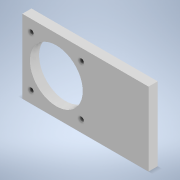
# Autodesk Inventor part: Stepper Plate
Saved by Autodesk Inventor 2020 (Build 240168000, 168)
## iProperties
Created: 2020-03-19
Part Number: Stepper Plate
Material: Generic
Document SubType Name: Modeling
Designer: DasNick
Density: 1 g/cm^3
Appearance: Default
Author: DasNick
Autodesk Inventor part; units mm, degrees
ref_plane "YZ Plane" through (0, 0, 0) normal (1, 0, 0) x (0, 1, 0)
ref_plane "XZ Plane" through (0, 0, 0) normal (0, 1, 0) x (-1, 0, 0)
ref_plane "XY Plane" through (0, 0, 0) normal (0, 0, 1) x (1, 0, 0)
sketch "Sketch1" plane through (0, 0, 0) normal (0, 0, 1) x (1, 0, 0)
  line L0 (-42.925, -19.7) -> (-38.525, -19.7) projected
  arc A0 (-38.525, -28.9) -> (-38.525, -19.7) centre (-38.525, -24.3) ccw projected
  line L1 (-38.525, -28.9) -> (-42.925, -28.9) projected
  line L2 (-42.925, -37.425) -> (-42.925, -28.9) projected
  arc A1 (-42.925, -37.425) -> (-37.425, -42.925) centre (-37.425, -37.425) ccw projected
  line L3 (19.7, -42.925) -> (-37.425, -42.925) projected
  line L4 (19.7, -42.925) -> (19.7, -38.525) projected
  arc A2 (28.9, -38.525) -> (19.7, -38.525) centre (24.3, -38.525) ccw projected
  line L5 (28.9, -38.525) -> (28.9, -42.925) projected
  line L6 (37.425, -42.925) -> (28.9, -42.925) projected
  arc A3 (37.425, -42.925) -> (42.925, -37.425) centre (37.425, -37.425) ccw projected
  line L7 (42.925, 19.7) -> (42.925, -37.425) projected
  line L8 (42.925, 19.7) -> (38.525, 19.7) projected
  arc A4 (38.525, 28.9) -> (38.525, 19.7) centre (38.525, 24.3) ccw projected
  line L9 (38.525, 28.9) -> (42.925, 28.9) projected
  line L10 (42.925, 37.425) -> (42.925, 28.9) projected
  arc A5 (42.925, 37.425) -> (37.425, 42.925) centre (37.425, 37.425) ccw projected
  line L11 (-19.7, 42.925) -> (37.425, 42.925) projected
  line L12 (-19.7, 42.925) -> (-19.7, 38.525) projected
  arc A6 (-28.9, 38.525) -> (-19.7, 38.525) centre (-24.3, 38.525) ccw projected
  line L13 (-28.9, 38.525) -> (-28.9, 42.925) projected
  line L14 (-37.425, 42.925) -> (-28.9, 42.925) projected
  arc A7 (-37.425, 42.925) -> (-42.925, 37.425) centre (-37.425, 37.425) ccw projected
  line L15 (-42.925, -19.7) -> (-42.925, 37.425) projected
  circle A8 centre (34.75, -34.75) radius 3.3 projected
  circle A9 centre (-34.75, -34.75) radius 3.3 projected
  circle A10 centre (34.75, 34.75) radius 3.3 projected
  circle A11 centre (-34.75, 34.75) radius 3.3 projected
  circle A12 centre (0, 0) radius 36.5125 projected
  line L16 (127.3875, 50.7471) -> (127.3875, -50.8529) projected
  line L17 (127.3875, 50.7471) -> (-47.0237, 50.7471)
  line L18 (-47.0237, 50.7471) -> (-47.0237, -50.8529)
  line L19 (-47.0237, -50.8529) -> (127.3875, -50.8529)
  point P0 (0, 0)
  dimension "d0" = 101.6
  constraints: 6 end point, 1 horizontal, 1 perpendicular
  measures "d0" distance of L17.end L18.end
extrude "Extrusion1" add sketch "Sketch1" along normal blind 12.7 contours L15 A7 L14 L13 A6 L12 L11 A5 L10 L9 A4 L8 L7 A3 L6 L5 A2 L4 L3 A1 L2 L1 A0 L0 | L16 L19 L18 L17
sketch "Sketch2" plane through (0, 0, 12.7) normal (0, 0, 1) x (1, 0, 0)
  line L0 (127.3875, -50.8529) -> (127.3875, 50.7471) projected
  line L1 (127.3875, 50.7471) -> (-47.0237, 50.7471) projected
  line L2 (-47.0237, 50.7471) -> (-47.0237, -50.8529) projected
  line L3 (-47.0237, -50.8529) -> (127.3875, -50.8529) projected
  circle A0 centre (0, 0) radius 36.5125 projected
  circle A1 centre (34.75, -34.75) radius 3.3 projected
  circle A2 centre (-34.75, 34.75) radius 3.3 projected
  circle A3 centre (34.75, 34.75) radius 3.3 projected
  circle A4 centre (-34.75, -34.75) radius 3.3 projected
  circle A5 centre (0, -0.6853) radius 9.525
  point P0 (0, 0)
  dimension "d3" = 19.05
  constraints: 1 centre point
  measures "d3" diameter of A5
extrude "Extrusion2" add sketch "Sketch2" against normal blind 9.525 contours A0
body "Solid1"
